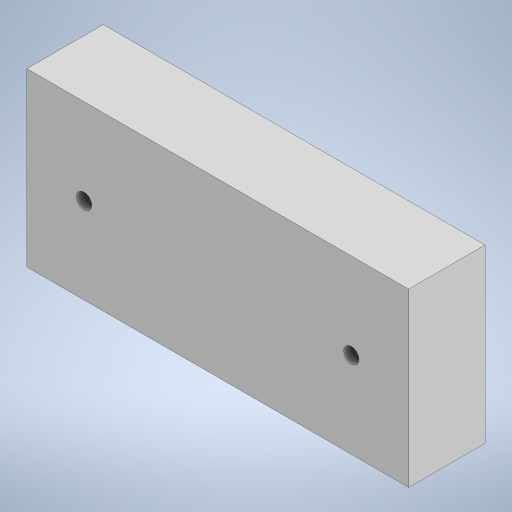
# Autodesk Inventor part: as3
Saved by Autodesk Inventor 2023 (Build 270158000, 158)
## iProperties
Created: 2022-12-05
Part Number: as3
Material: Generic
Document SubType Name: Modeling
Designer: daarn
Density: 1 g/cm^3
Appearance: Default
Author: daarn
Autodesk Inventor part; units mm, degrees
ref_plane "YZ Plane" through (0, 0, 0) normal (1, 0, 0) x (0, 1, 0)
ref_plane "XZ Plane" through (0, 0, 0) normal (0, 1, 0) x (-1, 0, 0)
ref_plane "XY Plane" through (0, 0, 0) normal (0, 0, 1) x (1, 0, 0)
sketch "Sketch1" plane through (0, 0, 0) normal (0, 0, 1) x (1, 0, 0)
  line L0 (0, 0) -> (100, 0)
  line L1 (100, 0) -> (100, -45)
  line L2 (100, -45) -> (0, -45)
  line L3 (0, -45) -> (0, 0)
  dimension "d0" = 100
  dimension "d1" = 45
  constraints: 8 end point, 2 parallel, 1 coincident, 1 horizontal, 1 perpendicular
  measures "d0" distance of L1.end L2.end
  measures "d1" distance of L0.end L1.end
extrude "Extrusion1" add sketch "Sketch1" along normal blind 20
sketch "Sketch2" plane through (0, 0, 0) normal (0, 0, -1) x (-1, 0, 0)
  point P0 (0, 0)
  point P1 (-15, -22.5)
  point P2 (-85, -22.5)
  dimension "d4" = 70
  dimension "d5" = 15
  dimension "d6" = 22.5
  constraints: 1 horizontal alignment
  measures "d4" distance of point (-85, -22.5) point (-15, -22.5)
  measures "d5" horizontal distance of point (0, 0) point (-15, -22.5)
  measures "d6" vertical distance of point (0, 0) point (-15, -22.5)
hole "Hole1" at (15, -22.5, 0) at (85, -22.5, 0) direction (0, 0, 1) diameter 4 depth 35 tip angle 118 counterbore diameter 8 counterbore depth 18
body "Solid1"
